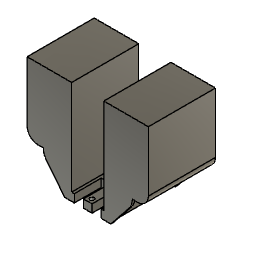
Load basket version 3 v4 (Autodesk Fusion 360 design; units mm, degrees)
Autodesk Fusion 360 part; units mm, degrees
note: some values were not read from the file. Chosen so that the rebuilt part matches the saved one: which bodies a step acts on. Set by a fixed rule: which sketch regions a step uses; which face or edge a step refers to.
sketch "Sketch1" plane through (0, 0, 0) normal (0, 0, 1) x (1, 0, 0)
  line L0 (0, 0) -> (66, 0)
  line L1 (66, 0) -> (66, 150)
  line L2 (66, 150) -> (0, 150)
  line L3 (0, 150) -> (0, 0)
  dimension "d3" = 150
  dimension "d4" = 66
  constraint horizontal L0
  constraint vertical L1
  constraint horizontal L2
  constraint vertical L3
  constraint coincident L0.start L3.end
  measures "d3" distance of L0.start L2.end
  measures "d4" distance of L0.start L0.end
extrude "Extrude1" add sketch "Sketch1" along normal blind 2 makes body 1
sketch "Sketch2" plane through (0, 0, 2) normal (0, 0, 1) x (-1, 0, 0)
  line L0 (0, -150) -> (0, 0)
  line L1 (0, 0) -> (-66, 0)
  line L2 (-66, 0) -> (-66, -150)
  line L3 (-66, -150) -> (0, -150)
  line L4 (0, 0) -> (-3, 0)
  line L5 (-3, 0) -> (-3, -150)
  line L6 (-3, -150) -> (0, -150)
  line L7 (0, -150) -> (0, 0)
  line L8 (-66, -150) -> (-63, -150)
  line L9 (-63, -150) -> (-63, 0)
  line L10 (-63, 0) -> (-66, 0)
  line L11 (-66, 0) -> (-66, -150)
  dimension "d5" = 3
  dimension "d6" = 3
  constraint horizontal L4
  constraint vertical L5
  constraint horizontal L6
  constraint vertical L7
  constraint coincident L3 L5.end
  constraint coincident L0.end L1.start
  constraint horizontal L8
  constraint vertical L9
  constraint horizontal L10
  constraint vertical L11
  constraint coincident L1 L9.end
  constraint coincident L2.end L3.start
  measures "d5" distance of L0.end L4.end
  measures "d6" distance of L2.end L8.end
extrude "Extrude2" add sketch "Sketch2" along normal blind 40 contours L0 L1 L3 L4 L5 L6 L7 | L1 L2 L3 L8 L9 L10 L11 bodies 1
extrude "Extrude3" add 1 faces at (0, 100, 28) along direction (-1, 0, 0) blind 60 on bodies 1 bodies 1
extrude "Extrude4" add 1 faces at (66, 50, 28) along direction (1, 0, 0) blind 60 on bodies 1 bodies 1
sketch "Sketch3" plane through (0, 0, 0) normal (0, 0, -1) x (1, 0, 0)
  line L0 (-60, -150) -> (126, -150)
  line L1 (126, -150) -> (126, 0)
  line L2 (126, 0) -> (-60, 0)
  line L3 (-60, 0) -> (-60, -150)
  line L4 (-50, -10) -> (0, -10)
  line L5 (0, -10) -> (0, -140)
  line L6 (0, -140) -> (-50, -140)
  line L7 (-50, -140) -> (-50, -10)
  constraint horizontal L4
  constraint vertical L5
  constraint horizontal L6
  constraint vertical L7
extrude "Extrude5" cut sketch "Sketch3" against normal blind 38 contours L4 L5 L6 L7 bodies 1
extrude "Extrude6" cut 1 faces at (-50, 96.6667, 12.6667) along direction (-1, 0, 0) blind 5 on bodies 1 bodies 1
extrude "Extrude7" add 1 faces at (0, 53.3333, 12.6667) along direction (-1, 0, 0) blind 2 on bodies 1 bodies 1
extrude "Extrude8" add 1 faces at (-60, 100, 28) along direction (-1, 0, 0) blind 20 on bodies 1 bodies 1
extrude "Extrude9" cut 1 faces at (-55, 96.6667, 12.6667) along direction (-1, 0, 0) blind 20 on bodies 1 bodies 1
extrude "Extrude10" add 1 faces at (-75, 96.6667, 12.6667) along direction (1, 0, 0) blind 1 on bodies 1 bodies 1
extrude "Extrude11" cut 1 faces at (-26, 10, 12.6667) along direction (0, -1, 0) blind 5 on bodies 1 bodies 1
extrude "Extrude12" cut 1 faces at (-26, 140, 12.6667) along direction (0, 1, 0) blind 5 on bodies 1 bodies 1
sketch "Sketch4" plane through (0, 0, 0) normal (0, 0, -1) x (1, 0, 0)
  line L0 (-74, -145) -> (-74, -5)
  line L1 (-74, -5) -> (-2, -5)
  line L2 (-2, -5) -> (-2, -145)
  line L3 (-2, -145) -> (-74, -145)
  line L4 (-80, -150) -> (126, -150)
  line L5 (126, -150) -> (126, 0)
  line L6 (126, 0) -> (-80, 0)
  line L7 (-80, 0) -> (-80, -150)
extrude "Extrude13" cut 1 faces at (-74, 51.6667, 25.3333) along direction (-1, 0, 0) blind 1 on bodies 1 bodies 1
extrude "Extrude14" add 1 faces at (43, 50, 2) along direction (0, 0, -1) blind 5 on bodies 1 bodies 1
extrude "Extrude15" add 1 faces at (43, 50, 2) along direction (0, 0, 1) blind 3 on bodies 1 bodies 1
sketch "Sketch5" plane through (0, 0, 0) normal (0, 0, -1) x (1, 0, 0)
  line L0 (-75, -5) -> (-2, -5)
  line L1 (-2, -5) -> (-2, -145)
  line L2 (-2, -145) -> (-75, -145)
  line L3 (-75, -145) -> (-75, -5)
  line L4 (3, -150) -> (3, 0)
  line L5 (3, 0) -> (-80, 0)
  line L6 (-80, 0) -> (-80, -150)
  line L7 (-80, -150) -> (3, -150)
  line L8 (63, -150) -> (68, -150)
  line L9 (68, -150) -> (68, -145)
  line L10 (68, -145) -> (141, -145)
  line L11 (141, -145) -> (141, -5)
  line L12 (141, -5) -> (68, -5)
  line L13 (68, -5) -> (68, -145)
  dimension "d35" = 5
  dimension "d36" = 73
  dimension "d37" = 140
  constraint perpendicular L1 L8
  constraint perpendicular L8 L9
  constraint horizontal L10
  constraint vertical L11
  constraint horizontal L12
  constraint vertical L13
  measures "d35" distance of L8.end L9.end
  measures "d36" distance of L9.end L10.end
  measures "d37" distance of L9.end L12.end
extrude "Extrude16" add 1 faces at (126, 50, 28) along direction (1, 0, 0) blind 25 on bodies 1 bodies 1
extrude "Extrude17" cut 1 faces at (151, 50, 28) along direction (-1, 0, 0) blind 5 on bodies 1 bodies 1
extrude "Extrude18" cut sketch "Sketch5" against normal blind 38 contours L10 L11 L12 L13 bodies 1
sketch "Sketch6" plane through (0, 0, -3) normal (0, 0, -1) x (1, 0, 0)
  line L0 (63, -150) -> (63, 0)
  line L1 (63, 0) -> (3, 0)
  line L2 (3, 0) -> (3, -150)
  line L3 (3, -150) -> (63, -150)
  line L4 (33, 0) -> (33, -8)
  line L5 (33, -8) -> (33, -142)
  line L6 (33, -142) -> (33, -150)
  circle A0 centre (33, -142) radius 4
  circle A1 centre (33, -8) radius 4
  dimension "d44" = 8
  dimension "d45" = 134
  dimension "d46" = 8
  dimension "d47" = 8
  constraint midpoint L1 L4.start
  constraint perpendicular L1 L4
  constraint perpendicular L1 L5
  constraint midpoint L3 L6.end
  constraint coincident L5.end L6.start
  constraint coincident L4.end L5.start
  measures "d44" distance of L4.start L4.end
  measures "d45" distance of L4.end L5.end
  measures "d46" diameter of A0
  measures "d47" diameter of A1
extrude "Extrude19" cut sketch "Sketch6" against normal blind 10 contours L5 L6 A0 | L5 L6 A0 | L4 L5 A1 | L4 L5 A1 bodies 1
sketch "Sketch7" plane through (0, 0, -3) normal (0, 0, -1) x (1, 0, 0)
  circle A0 centre (33, -142) radius 4
  circle A1 centre (33, -8) radius 4
  line L0 (63, -150) -> (63, 0)
  line L1 (63, 0) -> (3, 0)
  line L2 (3, 0) -> (3, -150)
  line L3 (3, -150) -> (63, -150)
  line L4 (63, -132.342) -> (58, -132.342)
  line L5 (33, -142) -> (33, -132)
  line L6 (33, -8) -> (33, -18)
  line L7 (58, -132) -> (8, -132)
  line L8 (8, -132) -> (8, -18)
  line L9 (8, -18) -> (58, -18)
  line L10 (58, -18) -> (58, -132)
  line L11 (33, -8) -> (33, 0)
  dimension "d50" = 5
  dimension "d51" = 10
  dimension "d52" = 10
  dimension "d53" = 50
  dimension "d54" = 114
  constraint coincident L0 L4.start
  constraint perpendicular L0 L4
  constraint coincident A0.centre L5.start
  constraint vertical L5
  constraint coincident A1.centre L6.start
  constraint vertical L6
  constraint horizontal L7
  constraint vertical L8
  constraint horizontal L9
  constraint vertical L10
  constraint midpoint L1 L11.end
  measures "d50" distance of L4.start L4.end
  measures "d51" distance of A0.centre L5.end
  measures "d52" distance of A1.centre L6.end
  measures "d53" distance of L7.start L7.end
  measures "d54" distance of L7.start L9.end
extrude "Extrude20" cut sketch "Sketch7" against normal blind 10 contours L7 L8 L9 L10 bodies 1
sketch "Sketch8" plane through (0, 150, 0) normal (0, 1, 0) x (-1, 0, 0)
  line L0 (-146, 42) -> (-146, 0)
  line L1 (-146, 0) -> (-63, 0)
  line L2 (-63, 0) -> (-63, -3)
  line L3 (-63, -3) -> (-3, -3)
  line L4 (-3, -3) -> (-3, 0)
  line L5 (-3, 0) -> (80, 0)
  line L6 (80, 0) -> (80, 42)
  line L7 (80, 42) -> (-3, 42)
  line L8 (-3, 42) -> (-3, 5)
  line L9 (-3, 5) -> (-63, 5)
  line L10 (-63, 5) -> (-63, 42)
  line L11 (-63, 42) -> (-146, 42)
  line L12 (80, 0) -> (-3, 0)
  line L13 (-3, 0) -> (-3, 42)
  line L14 (-3, 42) -> (80, 42)
  line L15 (80, 42) -> (80, 0)
  line L16 (-63, 42) -> (-146, 42)
  line L17 (-146, 42) -> (-146, 0)
  line L18 (-146, 0) -> (-63, 0)
  line L19 (-63, 0) -> (-63, 42)
  constraint horizontal L12
  constraint vertical L13
  constraint horizontal L14
  constraint vertical L15
  constraint coincident L7.end L8.start
  constraint coincident L5.end L6.start
  constraint horizontal L16
  constraint vertical L17
  constraint horizontal L18
  constraint vertical L19
  constraint coincident L0.end L1.start
  constraint coincident L10.end L11.start
extrude "Extrude21" add 1 faces at (-50.6667, 145, 25.3333) along direction (0, -1, 0) blind 25 on bodies 1 bodies 1
extrude "Extrude22" add 1 faces at (92.3333, 145, 25.3333) along direction (0, -1, 0) blind 25 on bodies 1 bodies 1
extrude "Extrude23" cut sketch "Sketch8" against normal blind 25 contours L0 L1 L10 L11 L16 L17 L18 L19 | L5 L6 L7 L8 L12 L13 L14 L15 bodies 1
extrude "Extrude41" cut 1 faces at (52.6518, 8.4679, -3) along direction (0, 0, 1) blind 3 on bodies 1 bodies 1
extrude "Extrude42" add 2 faces at (-24.6667, 83.3333, 42) (118.3333, 41.6667, 42) along direction (0, 0, 1) blind 100 on bodies 1 bodies 1
extrude "Extrude43" cut 2 faces at (92.3333, 43.3333, 38) (-50.6667, 43.3333, 38) along direction (0, 0, 1) blind 100 on bodies 1 bodies 1
sketch "Sketch16" plane through (0, 125, 0) normal (0, 1, 0) x (-1, 0, 0)
  line L0 (-3, 142) -> (-3, 5)
  line L1 (-3, 5) -> (-3, 0)
  line L2 (-3, 0) -> (80, 0)
  line L3 (80, 0) -> (80, 142)
  line L4 (80, 142) -> (-3, 142)
  line L5 (-3, 0) -> (10, 0)
  line L6 (10, 0) -> (50, 50)
  line L7 (50, 50) -> (80, 50)
  line L8 (-3, 0) -> (-3, 52.0463)
  constraint coincident L1.end L2.start
  constraint coincident L2 L5.end
  constraint perpendicular L1 L5
  constraint coincident L3 L7.end
  constraint perpendicular L3 L7
  constraint coincident L0 L8.end
extrude "Extrude44" cut sketch "Sketch16" against normal blind 1000 contours L2 L3 L6 L7 bodies 1
extrude "Extrude45" cut 1 faces at (-78.3333, 81.6667, 50) along direction (0, 0, 1) blind 10 on bodies 1 bodies 1
fillet "Fillet1" radius 20 1 edges at (-80, 62.5, 60) on bodies 1
fillet "Fillet2" radius 29 2 edges at (-50, 2.5, 50) (-50, 122.5, 50) on bodies 1
sketch "Sketch17" plane through (0, 150, 0) normal (0, 1, 0) x (-1, 0, 0)
  line L0 (-63, 0) -> (-3, 0)
  line L1 (-3, 0) -> (-3, 5)
  line L2 (-3, 5) -> (-63, 5)
  line L3 (-63, 5) -> (-63, 0)
  line L4 (-33, 0) -> (-163.9254, 0)
  line L5 (-163.9254, 0) -> (-163.9254, 153.2956)
  line L6 (-163.9254, 153.2956) -> (-33, 153.2956)
  line L7 (-33, 153.2956) -> (-33, 0)
  constraint horizontal L4
  constraint vertical L5
  constraint horizontal L6
  constraint vertical L7
  constraint midpoint L0 L4.start
extrude "Extrude46" cut sketch "Sketch17" against normal blind 1000 contours L0 L2 L3 L4 L7 | L2 L3 L4 L5 L6 L7 bodies 1
ref_plane "WorkPlane1" through (33, 135, 2.5) normal (1, 0, 0) x (0, 0, 1)
mirror "Mirror1" about plane through (33, 135, 2.5) normal (1, 0, 0) of bodies 1 merged
extrude "Extrude47" add 2 faces at (-24.6667, 83.3333, 142) (118.3333, 83.3333, 142) along direction (0, 0, 1) blind 50 on bodies 1 bodies 1
extrude "Extrude48" cut 2 faces at (-50.6667, 43.3333, 138) (116.6667, 43.3333, 138) along direction (0, 0, 1) blind 50 on bodies 1 bodies 1
extrude "Extrude49" add 1 faces at (13.3371, 8.567, 5) along direction (0, 0, 1) blind 10 on bodies 1 bodies 1
sketch "Sketch18" plane through (0, 132, 0) normal (0, -1, 0) x (1, 0, 0)
  line L0 (8, 15) -> (8, 0)
  line L1 (8, 0) -> (58, 0)
  line L2 (58, 0) -> (58, 15)
  line L3 (58, 15) -> (8, 15)
  line L4 (40, 0) -> (25, 0)
  line L5 (25, 0) -> (25, 15)
  line L6 (25, 15) -> (40, 15)
  line L7 (40, 15) -> (40, 0)
  constraint horizontal L4
  constraint vertical L5
  constraint horizontal L6
  constraint vertical L7
  constraint coincident L3 L5.end
  constraint coincident L1 L4.start
extrude "Extrude50" add sketch "Sketch18" along normal blind 114 contours L1 L3 L4 L5 L6 L7 bodies 1
extrude "Extrude51" cut 1 faces at (13.6667, 132, 5) along direction (0, 1, 0) blind 35 on bodies 1 bodies 1
extrude "Extrude52" cut 1 faces at (46, 132, 5) along direction (0, 1, 0) blind 45 on bodies 1 bodies 1
extrude "Extrude53" cut 2 faces at (19.3333, 18, 5) (52, 18, 5) along direction (0, -1, 0) blind 40 on bodies 1 bodies 1 makes body 2 at (63, 41.6667, 74) makes body 3 at (25, 100, 5)
sketch "Sketch19" plane through (25, 0, 0) normal (-1, 0, 0) x (0, -1, 0)
  line L0 (-150, 0) -> (0, 0)
  line L1 (0, 0) -> (0, 15)
  line L2 (0, 15) -> (-150, 15)
  line L3 (-150, 15) -> (-150, 0)
  line L4 (-50, 0) -> (-115, 0)
  line L5 (-115, 0) -> (-115, 15)
  line L6 (-115, 15) -> (-50, 15)
  line L7 (-50, 15) -> (-50, 0)
  constraint horizontal L4
  constraint vertical L5
  constraint horizontal L6
  constraint vertical L7
  constraint coincident L2 L5.end
  constraint coincident L0 L4.start
extrude "Extrude54" add sketch "Sketch19" along normal blind 20 and the other way blind 40 contours L0 L2 L4 L5 L6 L7 bodies 1 2 3
extrude "Extrude55" cut 2 faces at (6.3333, 150, 5) (61.3333, 150, 5) along direction (0, -1, 0) blind 25 on bodies 1 bodies 1
extrude "Extrude56" add 2 faces at (40, 138.3333, 5) (40, 33.3333, 10) along direction (1, 0, 0) blind 1 on bodies 1 bodies 1
extrude "Extrude57" add 1 faces at (-2, 43.3333, 62.6667) along direction (-1, 0, 0) blind 5 on bodies 1 bodies 1
extrude "Extrude58" add 1 faces at (68, 43.3333, 62.6667) along direction (1, 0, 0) blind 5 on bodies 1 bodies 1
